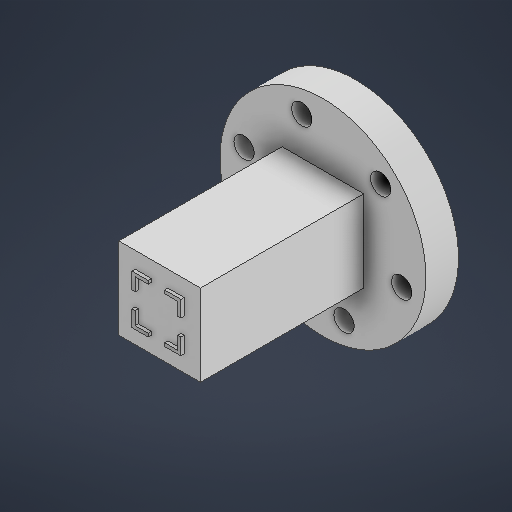
# Autodesk Inventor part: soporte p1
Saved by Autodesk Inventor 2026.1 (Build 301233020, 233B)
## iProperties
Created: 2026-01-16
Part Number: soporte p1
Material: Generic
Document SubType Name: Modeling
Designer: Marcelo
Density: 1 g/cm^3
Appearance: Default
Mass: 60.647 g
Surface Area: 141.001 cm^2
Volume: 60.647 cm^3
Author: Marcelo
Autodesk Inventor part; units mm, degrees
ref_plane "YZ Plane" through (0, 0, 0) normal (1, 0, 0) x (0, 1, 0)
ref_plane "XZ Plane" through (0, 0, 0) normal (0, 1, 0) x (-1, 0, 0)
ref_plane "XY Plane" through (0, 0, 0) normal (0, 0, 1) x (1, 0, 0)
sketch "Sketch1" plane through (0, 0, 0) normal (0, 0, 1) x (1, 0, 0)
  circle A0 centre (0, 0) radius 31.5
  line L0 (0, 0) -> (17.6777, 17.6777)
  line L1 (0, 0) -> (25, 0) construction
  circle A1 centre (17.6777, 17.6777) radius 3.1
  circle A2 centre (-6.4705, 24.1481) radius 3.1
  circle A3 centre (-24.1481, 6.4705) radius 3.1
  circle A4 centre (-17.6777, -17.6777) radius 3.1
  circle A5 centre (6.4705, -24.1481) radius 3.1
  circle A6 centre (24.1481, -6.4705) radius 3.1
  dimension "d0" = 63
  dimension "d1" = 25
  dimension "d2" = 45
  dimension "d3" = 6.2
  dimension "d6" = 360
  constraints: 7 centre point, 4 end point, 2 coincident, 1 equal length, 1 horizontal, 13 other
  measures "d0" diameter of A0
  measures "d1" distance of L0.start L0.end
  measures "d2" angle of L1 L0
  measures "d3" diameter of A1
extrude "Extrusion1" add sketch "Sketch1" along normal blind 10
sketch "Sketch2" plane through (0, 0, 10) normal (0, 0, 1) x (1, 0, 0)
  line L0 (12.5, -12.5) -> (-12.5, -12.5)
  line L1 (-12.5, -12.5) -> (-12.5, 12.5)
  line L2 (-12.5, 12.5) -> (12.5, 12.5)
  line L3 (12.5, 12.5) -> (12.5, -12.5)
  line L4 (12.5, -12.5) -> (-12.5, 12.5) construction
  line L5 (-12.5, -12.5) -> (12.5, 12.5) construction
  point P0 (0, 0)
  dimension "d10" = 25
  dimension "d11" = 25
  constraints: 12 end point, 2 midpoint, 2 parallel, 1 horizontal, 1 perpendicular
  measures "d10" distance of L1.end L2.end
  measures "d11" distance of L0.end L1.end
extrude "Extrusion2" add sketch "Sketch2" along normal blind 50
sketch "Sketch4" plane through (0, 0, 60) normal (0, 0, 1) x (1, 0, 0)
  line L0 (7.5, -7.5) -> (-7.5, -7.5)
  line L1 (-7.5, -7.5) -> (-7.5, 7.5)
  line L2 (-7.5, 7.5) -> (7.5, 7.5)
  line L3 (7.5, 7.5) -> (7.5, -7.5)
  line L4 (7.5, -7.5) -> (-7.5, 7.5) construction
  line L5 (-7.5, -7.5) -> (7.5, 7.5) construction
  line L6 (6.5, 6.5) -> (-6.5, 6.5)
  line L7 (-6.5, 6.5) -> (-6.5, -6.5)
  line L8 (-6.5, -6.5) -> (6.5, -6.5)
  line L9 (6.5, -6.5) -> (6.5, 6.5)
  line L10 (-9.4383, 2.5) -> (11.9316, 2.5)
  line L11 (-9.4383, -2.5) -> (9.2053, -2.5)
  line L12 (-2.5, 9.4032) -> (-2.5, -10.6036)
  line L13 (2.5, 9.4032) -> (2.5, -9.3606)
  point P0 (0, 0)
  point P1 (2.5, 7.5)
  point P2 (2.5, 6.5)
  point P3 (6.5, 2.5)
  point P4 (7.5, 2.5)
  point P5 (2.5, -6.5)
  point P6 (2.5, -7.5)
  point P7 (7.5, -2.5)
  point P8 (6.5, -2.5)
  point P9 (-2.5, -7.5)
  point P10 (-2.5, -6.5)
  point P11 (-6.5, -2.5)
  point P12 (-7.5, -2.5)
  point P13 (-2.5, 6.5)
  point P14 (-2.5, 7.5)
  point P15 (-7.5, 2.5)
  point P16 (-6.5, 2.5)
  dimension "d27" = 15
  dimension "d28" = 15
  dimension "d29" = 1
  dimension "d30" = 18.7639
  dimension "d31" = 5
  dimension "d32" = 5
  dimension "d33" = 5
  dimension "d34" = 5
  constraints: 28 end point, 4 parallel, 3 horizontal, 2 midpoint, 2 perpendicular, 2 vertical, 3 other
  measures "d27" distance of L1.end L2.end
  measures "d28" distance of L0.end L1.end
  measures "d29" distance between parallel lines of L2 L6
  measures "d30" distance of L13.start L13.end
  measures "d31" distance between parallel lines of L3 L13
  measures "d32" distance between parallel lines of L1 L12
  measures "d33" distance between parallel lines of L0 L11
  measures "d34" distance between parallel lines of L2 L10
extrude "Extrusion4" add sketch "Sketch4" along normal blind 1 contours L0 L13 L8 L9 L11 L3 | L0 L1 L11 L7 L8 L12 | L10 L9 L6 L13 L2 L3 | L1 L2 L12 L6 L7 L10
body "Solid1"
